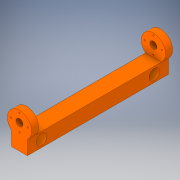
# Autodesk Inventor part: axil mount
Saved by Autodesk Inventor 2019 (Build 230136000, 136)
## iProperties
Created: 2019-03-12
Part Number: axil mount
Material: Generic
Document SubType Name: Modeling
Designer: Delta
Density: 1 g/cm^3
Appearance: Default(1)
Author: Delta
Autodesk Inventor part; units mm, degrees
ref_plane "YZ Plane" through (0, 0, 0) normal (1, 0, 0) x (0, 1, 0)
ref_plane "XZ Plane" through (0, 0, 0) normal (0, 1, 0) x (-1, 0, 0)
ref_plane "XY Plane" through (0, 0, 0) normal (0, 0, 1) x (1, 0, 0)
sketch "Sketch1" plane through (0, 0, 0) normal (0, 1, 0) x (-1, 0, 0)
  line L0 (0, 0) -> (14.351, 0)
  line L1 (14.351, 0) -> (14.351, -127)
  line L2 (14.351, -127) -> (0, -127)
  line L3 (0, -127) -> (0, 0)
  dimension "d0" = 127
  dimension "d1" = 14.351
  constraints: 8 end point, 2 parallel, 1 horizontal, 1 perpendicular
  measures "d0" distance of L0.end L1.end
  measures "d1" distance of L1.end L2.end
extrude "Extrusion1" add sketch "Sketch1" along normal blind 12.7
sketch "Sketch2" plane through (0, 0, 0) normal (1, 0, 0) x (0, 0, -1)
  circle A0 centre (12.7, 6.35) radius 4.7625
  circle A1 centre (114.3, 6.35) radius 4.7625
  line L0 (0, 12.7) -> (127, 12.7) projected
  line L1 (127, 0) -> (127, 12.7) projected
  point P0 (0, 0)
  dimension "d4" = 9.525
  dimension "d5" = 9.525
  dimension "d6" = 101.6
  dimension "d7" = 127
  dimension "d8" = 12.7
  dimension "d9" = 12.7
  dimension "d10" = 6.35
  dimension "d11" = 6.35
  constraints: 2 centre point
  measures "d4" diameter of A0
  measures "d5" diameter of A1
  measures "d6" distance of A0.centre A1.centre
  measures "d7" distance of L0.start L0.end
  measures "d8" distance from line of L1 A1.centre
  measures "d9" distance of L1.start L0.end
  measures "d10" distance from line of L0 A1.centre
  measures "d11" distance from line of L0 A0.centre
extrude "Extrusion2" cut sketch "Sketch2" against normal through all
sketch "Sketch3" plane through (-14.351, 0, 0) normal (0, 0, 1) x (1, 0, 0)
  line L0 (0, 12.7) -> (14.351, 12.7) projected
  circle A0 centre (7.1755, 22.3312) radius 9.525
  circle A1 centre (7.1755, 29.9512) radius 0.5953
  circle A2 centre (-0.4445, 22.3312) radius 0.5953
  circle A3 centre (14.7955, 22.3312) radius 0.5953
  circle A4 centre (7.1755, 14.7112) radius 0.5953
  line L1 (14.351, 0) -> (14.351, 12.7) projected
  line L2 (0, 0) -> (0, 12.7) projected
  arc A5 (14.351, 12.7) -> (0, 12.7) centre (7.1755, 20.9342) ccw
  circle A6 centre (7.1755, 22.3312) radius 3.175
  dimension "d15" = 19.05
  dimension "d16" = 1.1906
  dimension "d17" = 1.1906
  dimension "d18" = 1.1906
  dimension "d19" = 1.1906
  dimension "d20" = 7.62
  dimension "d28" = 0
  dimension "d29" = 10.922
  dimension "d32" = 6.35
  dimension "d33" = 7.62
  dimension "d34" = 7.62
  dimension "d35" = 7.62
  dimension "d36" = 0
  dimension "d37" = 9.6312
  dimension "d38" = 0
  dimension "d39" = 0
  dimension "d40" = 0
  constraints: 7 centre point, 2 point on circle, 1 coincident
  measures "d15" diameter of A0
  measures "d16" diameter of A1
  measures "d17" diameter of A2
  measures "d18" diameter of A4
  measures "d19" diameter of A3
  measures "d20" distance of A0.centre A3.centre
  measures "d28" horizontal distance between centres of A0 A5
  measures "d29" radius of A5
  measures "d32" diameter of A6
  measures "d33" distance of A0.centre A1.centre
  measures "d34" distance of A2.centre A0.centre
  measures "d35" distance of A0.centre A4.centre
  measures "d36" vertical distance of A2.centre A6.centre
  measures "d37" distance from line of L0 A6.centre
  measures "d38" horizontal distance of A4.centre A0.centre
  measures "d39" vertical distance of A0.centre A3.centre
  measures "d40" horizontal distance of A1.centre A0.centre
ref_plane "Work Plane1" through (-14.351, 0, -63.5) normal (0, 0, 1) x (1, 0, 0)
extrude "Extrusion4" add sketch "Sketch3" against normal blind 6.35 contours A0 | A5 L0
mirror "Mirror1" about plane through (-14.351, 0, -63.5) normal (0, 0, 1) of "Extrusion4"
equation "\"d5\" = d4"
equation "\"d8\" = -0.5 * d6 + 0.5 * d7"
equation "\"d10\" = 0.5 * d9"
equation "\"d11\" = d10"
equation "\"d17\" = d16"
equation "\"d18\" = d17"
equation "\"d19\" = d17"
body "Solid1"
